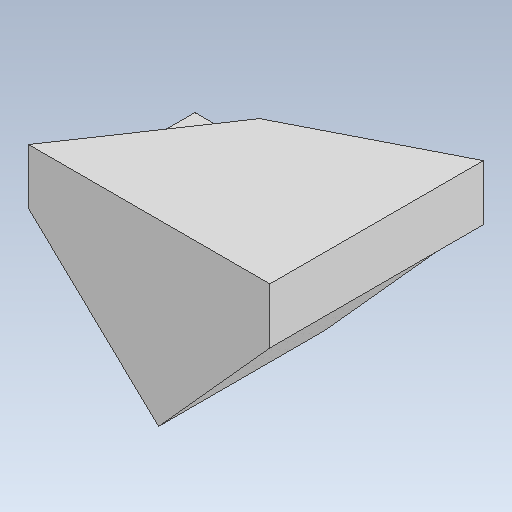
# Autodesk Inventor part: secure_to_hoop_machined
Saved by Autodesk Inventor 2021 (Build 250183000, 183)
## iProperties
Created: 2021-06-08
Part Number: secure_to_hoop_machined
Material: Generic
Document SubType Name: Modeling
Density: 1 g/cm^3
Appearance: Default
Autodesk Inventor part; units mm, degrees
ref_plane "YZ Plane" through (0, 0, 0) normal (1, 0, 0) x (0, 1, 0)
ref_plane "XZ Plane" through (0, 0, 0) normal (0, 1, 0) x (-1, 0, 0)
ref_plane "XY Plane" through (0, 0, 0) normal (0, 0, 1) x (1, 0, 0)
sketch "Sketch1" plane through (0, 0, 0) normal (0, 1, 0) x (-1, 0, 0)
  line L0 (0, 0) -> (43.506, 0)
  line L1 (0, -38.4908) -> (0, 0)
  line L2 (43.506, 0) -> (26.7302, -24.8711)
  line L3 (26.7302, -24.8711) -> (0, -38.4908)
  dimension "d0" = 56
  dimension "d2" = 30
  dimension "d3" = 30
  dimension "d10" = 27
  constraints: 8 end point, 2 point on line, 1 horizontal, 1 perpendicular
  measures "d0" angle of L2 L0
  measures "d2" distance of L0.end L2.end
  measures "d3" distance of L2.end L1.start
  measures "d10" angle of L0 L3
extrude "Extrusion1" add sketch "Sketch1" along normal blind 10
sketch "Sketch2" plane through (0, 0, 0) normal (0, 0, 1) x (1, 0, 0)
  line L0 (0, 0) -> (-20.0739, -22.2943)
  line L1 (-43.506, 0) -> (0, 0) projected
  line L2 (-26.7302, 0) -> (-43.506, 0) projected
  line L3 (-20.0739, -22.2943) -> (-43.506, 0)
  line L4 (0, 0) -> (-26.7302, 0) projected
  line L5 (-43.506, 0) -> (0, 0)
  dimension "d6" = 48
  dimension "d7" = 30
  constraints: 6 end point, 1 collinear
  measures "d6" angle of L1 L0
  measures "d7" distance of L0.start L0.end
extrude "Extrusion2" add sketch "Sketch2" against normal blind 30
equation "\"d2\" = secure_arm_thickness"
equation "\"d3\" = d2"
equation "\"d7\" = secure_arm_thickness"
equation "\"d8\" = secure_arm_hold_thickness"
equation "\"hoop_angle_z\" = 45deg"
equation "\"hoop_bearing_length\" = 5deg"
equation "\"hoop_cable_diam\" = 5"
equation "\"hoop_cable_pulley_diam\" = 22"
equation "\"hoop_thickness_large\" = 4"
equation "\"hoop_thickness_medium\" = 3.2"
equation "\"hoop_thickness_small\" = 2"
equation "\"hoop_width_large\" = 51"
equation "\"hoop_width_medium\" = 33.7"
equation "\"hoop_width_small\" = 25.4"
equation "\"rack_tooth_addendum\" = 5"
equation "\"rack_tooth_dedendum\" = 5"
equation "\"rack_tooth_thickness\" = 5"
equation "\"secure_arm_angle\" = 35deg"
equation "\"secure_arm_hold_thickness\" = 30"
equation "\"secure_arm_radii\" = 9"
equation "\"secure_arm_thickness\" = 30"
equation "\"support_baseClamp_platformLengthBuffer\" = 35"
equation "\"support_baseClamp_platformThickness\" = 15"
equation "\"support_baseClamp_platformWidthBuffer\" = 0"
equation "\"support_baseClamp_sleeveHoleDiameter\" = 12"
equation "\"support_baseClamp_sleeveSweepTerminationAngle\" = 55deg"
equation "\"support_baseClamp_thickness\" = 8"
equation "\"support_frame_endHoleBuffer\" = 25"
equation "\"support_frame_squareBarFillet\" = 2"
equation "\"support_frame_squareBarThickness\" = 5"
equation "\"hoop_tabs_thickness\" = 6"
equation "\"hoop_tabs_hole\" = 12"
equation "\"wheelchair_deployed_width\" = 635"
equation "\"wheelchair_deployed_length\" = 1067"
equation "\"wheelchair_deployed_height\" = 914"
equation "\"sm_varx_squareBarThickness\" = 2.5"
equation "\"sm_varx_pinPlate_thickness\" = 5"
equation "\"sm_varx_pinPlate_holeDiameter\" = 5"
equation "\"sm_varx_member_tolerance\" = 0.5"
equation "\"hoop_bushing23_radialInterference\" = 0"
equation "\"hoop_bushing12_radialInterference\" = 0"
equation "\"hoop_bushing12_od\" = -2 * hoop_thickness_large + hoop_width_large + hoop_bushing12_radialInterference"
equation "\"hoop_bushing23_od\" = -2 * hoop_thickness_medium + hoop_width_medium + hoop_bushing23_radialInterference"
body "Solid1"
